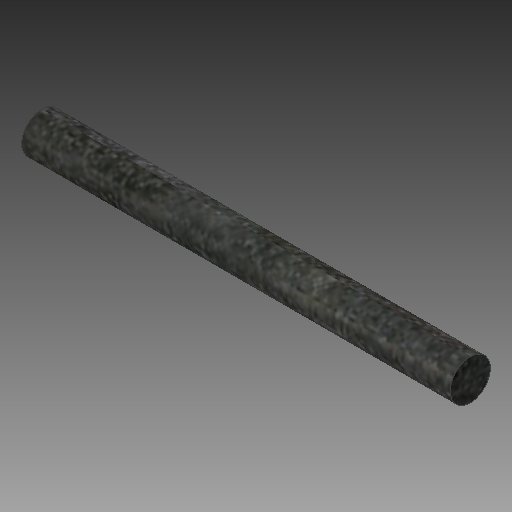
# Autodesk Inventor part: InnerTubeStopPost
Saved by Autodesk Inventor 2017 (Build 210142000, 142)
## iProperties
Created: 2016-02-17
Part Number: InnerTubeStopPost
Material: Steel
Document SubType Name: Modeling
Designer: steele
Density: 7.85 g/cm^3
Appearance: Plate
Mass: 56.8307 g
Surface Area: 31.8276 cm^2
Volume: 7.23958 cm^3
Author: steele
Autodesk Inventor part; units mm, degrees
ref_plane "YZ Plane" through (0, 0, 0) normal (1, 0, 0) x (0, 1, 0)
ref_plane "XZ Plane" through (0, 0, 0) normal (0, 1, 0) x (-1, 0, 0)
ref_plane "XY Plane" through (0, 0, 0) normal (0, 0, 1) x (1, 0, 0)
sketch "Sketch1" plane through (0, 0, 0) normal (1, 0, 0) x (0, 1, 0)
  circle A0 centre (0, 0) radius 4.7625
  dimension "d0" = 9.525
  constraints: 1 centre point, 1 coincident
  measures "d0" diameter of A0
extrude "Extrusion1" add sketch "Sketch1" along normal mid plane 101.6
equation "\"d0\" = diam"
equation "\"d1\" = length"
equation "\"diam\" = 9.525"
equation "\"length\" = 101.6"
body "Solid1"
